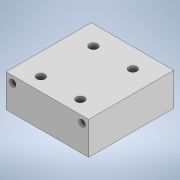
# Autodesk Inventor part: Palm Spacer
Saved by Autodesk Inventor 2021 (Build 250183000, 183)
## iProperties
Created: 2022-09-22
Part Number: Palm Spacer
Material: Generic
Document SubType Name: Modeling
Designer: ereg140
Density: 1 g/cm^3
Appearance: Default
Author: ereg140
Autodesk Inventor part; units mm, degrees
ref_plane "YZ Plane" through (0, 0, 0) normal (1, 0, 0) x (0, 1, 0)
ref_plane "XZ Plane" through (0, 0, 0) normal (0, 1, 0) x (-1, 0, 0)
ref_plane "XY Plane" through (0, 0, 0) normal (0, 0, 1) x (1, 0, 0)
sketch "Sketch1" plane through (0, 0, 0) normal (0, 1, 0) x (-1, 0, 0)
  line L0 (12.5625, -13.9) -> (-12.5625, -13.9)
  line L1 (-12.5625, -13.9) -> (-12.5625, 12)
  line L2 (-12.5625, 12) -> (12.5625, 12)
  line L3 (12.5625, 12) -> (12.5625, -13.9)
  circle A0 centre (6, -8) radius 1.25
  circle A1 centre (-6, -8) radius 1.25
  circle A2 centre (6, 8) radius 1.25
  circle A3 centre (-6, 8) radius 1.25
  point P0 (0, 0)
  point P1 (0, -13.9)
  dimension "d1" = 2.5
  dimension "d2" = 2.5
  dimension "d3" = 2.5
  dimension "d4" = 2.5
  dimension "d5" = 5.9
  dimension "d6" = 12
  dimension "d7" = 16
  dimension "d8" = 6
  dimension "d9" = 8
  dimension "d10" = 4
  dimension "d11" = 25.125
  constraints: 8 end point, 4 centre point, 3 vertical alignment, 2 horizontal alignment, 2 parallel, 1 horizontal, 1 midpoint, 1 perpendicular
  measures "d1" diameter of A0
  measures "d2" diameter of A1
  measures "d3" diameter of A2
  measures "d4" diameter of A3
  measures "d5" distance from line of L0 A0.centre
  measures "d6" distance of A1.centre A0.centre
  measures "d7" distance of A0.centre A2.centre
  measures "d8" horizontal distance of point (0, 0) A0.centre
  measures "d9" vertical distance of point (0, 0) A2.centre
  measures "d10" distance from line of A2.centre L2
  measures "d11" distance between parallel lines of L1 L3
extrude "Extrusion1" add sketch "Sketch1" along normal blind 10
sketch "Sketch2" plane through (12.5625, 0, -13.9) normal (0, 0, -1) x (-1, 0, 0)
  circle A0 centre (2, 8) radius 1
  circle A1 centre (23.125, 8) radius 1
  line L0 (0, 10) -> (25.125, 10) projected
  point P0 (12.5625, 0)
  dimension "d14" = 21.125
  dimension "d15" = 10.5625
  dimension "d16" = 2
  dimension "d17" = 2
  dimension "d18" = 2
  constraints: 2 centre point, 1 horizontal alignment
  measures "d14" distance of A1.centre A0.centre
  measures "d15" horizontal distance of point (12.562, 0) A0.centre
  measures "d16" diameter of A0
  measures "d17" diameter of A1
  measures "d18" distance from line of L0 A0.centre
extrude "Extrusion2" cut sketch "Sketch2" against normal through all
equation "\"d4\" = d2"
equation "\"d8\" = 0.5 * d6"
equation "\"d9\" = 0.5 * d7"
equation "\"d15\" = 0.5 * d14"
body "Solid1"
